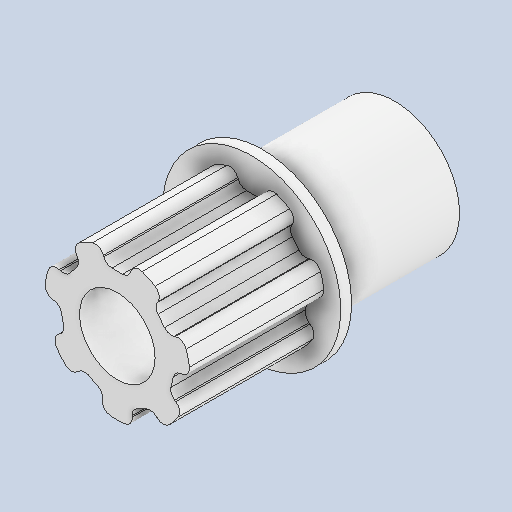
# Autodesk Inventor part: 동기식 풀리1
Saved by Autodesk Inventor 2025.3 (Build 293356030, 356C)
## iProperties
CustomPartVersion: 1
Created: 2025-09-07
Part Number: 동기식 풀리1
Material: PLA+ filament
Document SubType Name: Modeling
Designer: MSI
Density: 1.23 g/cm^3
Appearance: 일반
Mass: 20.0273 g
Surface Area: 81.6332 cm^2
Volume: 16.2823 cm^3
Author: MSI
Autodesk Inventor part; units mm, degrees
ref_plane "YZ Plane" through (0, 0, 0) normal (1, 0, 0) x (0, 1, 0)
ref_plane "XZ Plane" through (0, 0, 0) normal (0, 1, 0) x (-1, 0, 0)
ref_plane "XY Plane" through (0, 0, 0) normal (0, 0, 1) x (1, 0, 0)
sketch "풀리 스케치" plane through (0, 0, 0) normal (0, 0, 1) x (1, 0, 0)
  circle A0 centre (0, 0) radius 14.1489 construction
  circle A1 centre (0, 0) radius 13.4631
  circle A2 centre (0, 0) radius 10.4151
  line L0 (-3.0753, 13.1071) -> (-2.0955, 10.4151)
  line L1 (-2.0955, 10.4151) -> (2.0955, 10.4151)
  line L2 (2.0955, 10.4151) -> (3.0753, 13.1071)
  line L3 (0, 0) -> (0, 13.4631) construction
  point P0 (0, 10.4151)
  dimension "d0" = 28.2978
  dimension "d1" = 0.6858
  dimension "d2" = 3.048
  dimension "d3" = 40
  dimension "d4" = 4.191
  constraints: 8 end point, 3 coincident, 3 point on circle, 2 centre point, 1 horizontal, 1 midpoint, 1 point on line, 1 vertical, 1 vertical alignment, 3 other
  measures "d0" diameter of A0
  measures "d1" radial gap between concentric circles of A0 A1
  measures "d3" angle of L2 L0
  measures "d4" distance of L0.end L1.end
extrude "기본 본체" add sketch "풀리 스케치" along normal mid plane 24.892 contours A2 | A1 L0 L1 L2 | L2 L1 L0 A1
extrude "톱니" cut sketch "풀리 스케치" along normal through all both and the other way through all contours L2 L1 L0 A1 picked at (-1.0429, 11.4179)
fillet "Fillet" radius 1.6002 2 edges at (2.0955, 10.4151, 0) (-2.0955, 10.4151, 0)
fillet "Fillet" radius 1.6002 4 edges at (-3.0753, 13.1071, 6.223) (-3.0753, 13.1071, -6.223) (3.0753, 13.1071, 6.223) (3.0753, 13.1071, -6.223)
pattern_circular "Teeth" count 7 over 360 about axis through (0, 0, -10) along (0, 0, 1) of "톱니", "Fillet"
feature "왼쪽 플랜지" [suppressed]
feature "오른쪽 플랜지" [suppressed]
sketch "스케치2" plane through (0, 0, 12.446) normal (0, 0, 1) x (1, 0, 0)
  circle A0 centre (0, 0) radius 7
  dimension "d17" = 14
  constraints: 1 centre point, 1 coincident
  measures "d17" diameter of A0
extrude "돌출3" cut sketch "스케치2" against normal through all
sketch "스케치3" plane through (0, 0, -12.446) normal (0, 0, -1) x (-1, 0, 0)
  circle A0 centre (0, 0) radius 16.5
  circle A1 centre (0, 0) radius 7 projected
  dimension "d20" = 33
  constraints: 1 centre point, 1 coincident
  measures "d20" diameter of A0
extrude "돌출4" add sketch "스케치3" along normal blind 2
sketch "스케치4" plane through (0, 0, -14.446) normal (0, 0, -1) x (-1, 0, 0)
  circle A0 centre (0, 0) radius 7 projected
  circle A1 centre (0, 0) radius 12
  dimension "d23" = 5
  constraints: 1 centre point
  measures "d23" radial gap between concentric circles of A0 A1
extrude "돌출5" add sketch "스케치4" along normal blind 24.5
equation "\"d1\" = da_a"
equation "\"d2\" = da_hg"
equation "\"d3\" = 2 * da_fi"
equation "\"d4\" = da_bw"
equation "\"d5\" = da_bf"
equation "\"d7\" = da_bf"
equation "\"d9\" = da_rb"
equation "\"d10\" = da_rt"
equation "\"da_pb\" = 12.7"
equation "\"da_fi\" = 20deg"
equation "\"da_hg\" = 3.048"
equation "\"da_bw\" = 4.191"
equation "\"da_rb\" = 1.6002"
equation "\"da_rt\" = 1.6002"
equation "\"da_a\" = 0.6858"
equation "\"da_bf\" = 24.892"
equation "\"da_wf\" = 1.5"
equation "\"da_hf\" = 1.5"
body "Solid1"
